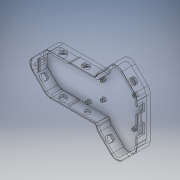
# Autodesk Inventor part: Arduino simple 4 channel ttl bottom Mega
Saved by Autodesk Inventor 2017 (Build 210142000, 142)
## iProperties
Created: 2016-10-03
Part Number: Arduino simple 4 channel ttl bottom Mega
Material: Generic
Document SubType Name: Modeling
Designer: andrew
Density: 1 g/cm^3
Appearance: Default
Author: andrew
Autodesk Inventor part; units mm, degrees
(part 1 of 2)
ref_plane "YZ Plane" through (0, 0, 0) normal (1, 0, 0) x (0, 1, 0)
ref_plane "XZ Plane" through (0, 0, 0) normal (0, 1, 0) x (-1, 0, 0)
ref_plane "XY Plane" through (0, 0, 0) normal (0, 0, 1) x (1, 0, 0)
sketch "Sketch1" plane through (0, 0, 0) normal (0, 1, 0) x (-1, 0, 0)
  circle A0 centre (66.1, -35.5) radius 2.345
  circle A1 centre (15.3, -50.7) radius 2.345
  circle A2 centre (14, -2.5) radius 2.345
  circle A3 centre (66.1, -7.6) radius 2.345
  line L0 (0, 0) -> (68.6, 0) construction
  line L1 (0, -53.3) -> (0, 0) construction
  line L2 (66.1, -53.3) -> (0, -53.3) construction
  line L3 (66.1, -40.6) -> (66.1, -53.3) construction
  line L4 (68.6, -40.6) -> (66.1, -40.6) construction
  line L5 (68.6, 0) -> (68.6, -40.6) construction
  line L6 (0, -12.2) -> (0, -3.3) construction
  line L7 (-1.8, -3.3) -> (0, -3.3) construction
  line L8 (-1.8, -12.2) -> (-1.8, -3.3) construction
  line L9 (0, -12.2) -> (-1.8, -12.2) construction
  line L10 (-6.2, -43.5895) -> (-6.2, -31.5895) construction
  line L11 (0, -43.5895) -> (0, -31.5895) construction
  line L12 (-6.2, -31.5895) -> (0, -31.5895) construction
  line L13 (-6.2, -43.5895) -> (-6.2, -31.5895) construction
  line L14 (0, -43.5895) -> (-6.2, -43.5895) construction
  circle A4 centre (14, -2.5) radius 1.6
  circle A5 centre (15.3, -50.7) radius 1.6
  circle A6 centre (66.1, -35.5) radius 1.6
  circle A7 centre (66.1, -7.6) radius 1.6
  line L15 (66.1, -35.5) -> (90.2, -35.5) construction
  line L16 (14, -2.5) -> (-6.2, -2.5) construction
  line L17 (0, -2.5) -> (96.52, -2.5) construction
  line L18 (0, -2.5) -> (96.52, -2.5) construction
  line L19 (90.2, -35.5) -> (90.2, -50.7) construction
  circle A8 centre (90.2, -50.7) radius 1.6
  circle A9 centre (90.2, -50.7) radius 2.345
  circle A10 centre (96.52, -2.5) radius 1.6
  circle A11 centre (96.52, -2.5) radius 2.345
  line L20 (68.6, -20.3) -> (101.6, -20.3) construction
  line L21 (101.6, -20.3) -> (101.6, 10.1637) construction
  dimension "d223" = 14
  dimension "d224" = 66.1
  dimension "d225" = 2.5
  dimension "d226" = 7.6
  dimension "d227" = 35.5
  dimension "d228" = 50.7
  dimension "d229" = 24.1
  dimension "d230" = 96.52
  dimension "d231" = 0
  dimension "d232" = 15.2
  dimension "d234" = 33
  constraints: 44 end point, 12 centre point, 4 horizontal, 2 collinear, 2 point on line, 2 vertical, 1 midpoint
  measures "d223" distance from line of L1 L16.start
  measures "d224" distance from line of A7.centre L1
  measures "d225" distance from line of L0 A2.centre
  measures "d226" distance from line of L0 A7.centre
  measures "d227" distance from line of L0 A0.centre
  measures "d228" distance from line of L0 A5.centre
  measures "d229" distance of L15.start L15.end
  measures "d230" distance of L17.start L17.end
  measures "d231" distance between parallel lines of L17 L18
  measures "d232" distance of L15.end L19.end
  measures "d234" distance of L20.start L20.end
extrude "Extrusion1" add sketch "Sketch1" along normal blind 4.69
draft "FaceDraft1" angle 10 pull direction (0, -1, 0) faces at (-68.4146, 3.1267, -7.9762) (-64.2253, 3.1267, -36.9087) (-16.3146, 3.1267, -2.8762) (-17.6146, 3.1267, -51.0762) (-98.8346, 3.1267, -2.8762) (-92.5146, 3.1267, -51.0762) fixed edges at (-63.755, 0, -7.6) (-63.755, 0, -35.5) (-11.655, 0, -2.5) (-12.955, 0, -50.7) (-94.175, 0, -2.5) (-87.855, 0, -50.7)
sketch "Sketch2" plane through (-66.1, 4.69, -7.6) normal (0, 1, 0) x (1, 0, 0)
  circle A0 centre (0.0002, 27.8999) radius 2.345 construction
  circle A1 centre (50.8002, 43.0999) radius 2.345 construction
  circle A2 centre (52.1002, -5.1001) radius 2.345 construction
  circle A3 centre (0.0002, -0.0001) radius 2.345 construction
  line L0 (66.1002, -7.6001) -> (-2.4998, -7.6001) construction
  line L1 (66.1002, 45.6999) -> (66.1002, -7.6001) construction
  line L2 (0.0002, 45.6999) -> (66.1002, 45.6999) construction
  line L3 (0.0002, 32.9999) -> (0.0002, 45.6999) construction
  line L4 (-2.4998, 32.9999) -> (0.0002, 32.9999) construction
  line L5 (-2.4998, -7.6001) -> (-2.4998, 32.9999) construction
  line L6 (66.1002, 4.5999) -> (66.1002, -4.3001) construction
  line L7 (67.9002, -4.3001) -> (66.1002, -4.3001) construction
  line L8 (66.1002, 4.5999) -> (67.9002, 4.5999) construction
  line L9 (72.3002, 35.9894) -> (72.3002, 23.9894) construction
  line L10 (66.1002, 35.9894) -> (66.1002, 23.9894) construction
  line L11 (72.3002, 23.9894) -> (66.1002, 23.9894) construction
  line L12 (72.3002, 35.9894) -> (72.3002, 23.9894) construction
  line L13 (66.1002, 35.9894) -> (72.3002, 35.9894) construction
  circle A4 centre (52.1002, -5.1001) radius 1.6 construction
  circle A5 centre (50.8002, 43.0999) radius 1.6 construction
  circle A6 centre (0.0002, 27.8999) radius 1.6 construction
  circle A7 centre (0.0002, -0.0001) radius 1.6 construction
  line L14 (-4.4998, -9.6001) -> (68.1002, -9.6001) construction
  line L15 (-1.9998, 47.6999) -> (-1.9998, 34.9999) construction
  line L16 (-1.9998, 34.9999) -> (-4.4998, 34.9999) construction
  line L17 (66.1002, 4.5999) -> (74.6809, 4.5999) construction
  line L18 (74.6809, 4.5999) -> (74.6809, -4.3001) construction
  line L19 (74.6809, -4.3001) -> (66.1002, -4.3001) construction
  line L20 (66.1002, -4.3001) -> (66.1002, 4.5999) construction
  line L21 (66.1002, 23.9894) -> (80.0982, 23.9894) construction
  line L22 (80.0982, 23.9894) -> (80.0982, 35.9894) construction
  line L23 (80.0982, 35.9894) -> (66.1002, 35.9894) construction
  line L24 (66.1002, 35.9894) -> (66.1002, 23.9894) construction
  line L25 (76.0853, 6.0043) -> (64.6958, 6.0043) construction
  line L26 (64.6958, 6.0043) -> (64.6958, -5.7045) construction
  line L27 (64.6958, -5.7045) -> (76.0853, -5.7045) construction
  line L28 (76.0853, -5.7045) -> (76.0853, 6.0043) construction
  line L29 (82.0982, 21.9894) -> (64.1002, 21.9894) construction
  line L30 (64.1002, 21.9894) -> (64.1002, 37.9894) construction
  line L31 (64.1002, 37.9894) -> (82.0982, 37.9894) construction
  line L32 (82.0982, 37.9894) -> (82.0982, 21.9894) construction
  line L33 (68.1002, 6.0043) -> (71.1002, 6.0043)
  line L34 (71.1002, 21.9894) -> (68.1002, 21.9894)
  line L35 (71.1002, 37.9894) -> (68.1002, 37.9894) construction
  line L36 (68.1002, 6.0043) -> (68.1002, 47.6999) construction
  line L37 (68.1002, 47.6999) -> (68.1002, 37.9894) construction
  line L38 (68.1002, 21.9894) -> (68.1002, 6.0043)
  line L39 (71.1002, 37.9894) -> (71.1002, 50.6999) construction
  line L40 (68.1002, -9.6001) -> (68.1002, -10.3919) construction
  line L41 (68.1002, 47.6999) -> (68.1002, 49.1999) construction
  line L42 (68.1002, 47.6999) -> (69.6002, 47.6999) construction
  line L43 (71.1002, 50.6999) -> (71.1002, 52.1999) construction
  line L44 (71.1002, 50.6999) -> (72.6002, 50.6999) construction
  line L45 (6.3002, -11.1001) -> (-38.5071, -11.1001)
  line L46 (71.1002, -14.1001) -> (71.1002, -5.7045) construction
  line L47 (71.1002, 6.0043) -> (71.1002, 21.9894)
  line L48 (71.1002, -5.7045) -> (68.1002, -5.7045) construction
  line L49 (-74.3828, 65.0749) -> (-74.3828, 33.3249) construction
  line L50 (-62.8828, 49.1999) -> (-62.8828, 33.3249) construction
  line L51 (-67.8378, 49.1999) -> (-62.8828, 49.1999) construction
  line L52 (-67.8378, 33.3249) -> (-67.8378, 65.0749) construction
  line L53 (-74.3828, 33.3249) -> (-61.2928, 33.3249) construction
  line L54 (-74.3828, 49.1999) -> (-61.2928, 49.1999) construction
  line L55 (-68.9958, 47.6999) -> (-42.4924, 47.6999)
  line L56 (-62.8828, 33.3249) -> (-72.7928, 33.3249) construction
  line L57 (-86.1418, 1.9038) -> (-89.6456, 5.4076) construction
  line L58 (-89.6456, 5.4076) -> (-78.4202, 16.6329) construction
  line L59 (-78.4202, 16.6329) -> (-71.4128, 9.6254) construction
  line L60 (-79.5445, 17.7572) -> (-70.2885, 8.5011) construction
  line L61 (-101.9952, -4.6935) -> (-79.5445, 17.7572) construction
  line L62 (-90.7699, 6.5319) -> (-81.5138, -2.7242) construction
  line L63 (-71.4128, 9.6254) -> (-82.6381, -1.5999) construction
  line L64 (-75.0062, -7.1105) -> (-95.1562, 13.0395)
  line L65 (-74.9165, 13.1292) -> (-97.3672, -9.3215) construction
  line L66 (-78.1882, -10.2925) -> (-98.3382, 9.8575)
  line L67 (-70.2885, 8.5011) -> (-92.7391, -13.9495) construction
  line L68 (-92.7391, -13.9495) -> (-101.9952, -4.6935) construction
  arc A8 (-98.3382, 28.2423) -> (-98.3382, 9.8575) centre (-89.1458, 19.0499) ccw
  arc A9 (-95.1562, 25.0603) -> (-95.1562, 13.0395) centre (-89.1458, 19.0499) ccw
  line L69 (-42.4924, -9.6001) -> (-68.9958, -9.6001)
  arc A10 (-75.0062, -7.1105) -> (-68.9958, -9.6001) centre (-68.9958, -1.1001) ccw
  arc A11 (-78.1882, -10.2925) -> (-68.9958, -14.1001) centre (-68.9958, -1.1001) ccw
  line L70 (-61.2928, 33.3249) -> (-61.2928, 65.0749) construction
  line L71 (-72.7928, 33.3249) -> (-72.7928, 49.1999) construction
  arc A12 (-68.9958, 47.6999) -> (-75.0062, 45.2103) centre (-68.9958, 39.1999) ccw
  arc A13 (-68.9958, 52.1999) -> (-78.1882, 48.3923) centre (-68.9958, 39.1999) ccw
  line L72 (-98.3382, 28.2423) -> (-78.1882, 48.3923)
  line L73 (-95.1562, 25.0603) -> (-75.0062, 45.2103)
  line L74 (-40.4998, -10.3501) -> (-40.4998, -10.3501)
  line L75 (-40.4998, 48.4499) -> (-40.4998, 48.4499)
  line L76 (-40.3711, -10.4788) -> (-40.6284, -10.2214)
  line L77 (-40.3711, 48.5786) -> (-39.7498, 49.1999)
  line L78 (-85.0812, 2.9645) -> (-92.329, 10.2123) construction
  line L79 (-92.329, 10.2123) -> (-92.329, 27.8875) construction
  line L80 (-35.4998, 19.0499) -> (-68.4998, 19.0499) construction
  line L81 (8.5832, -108.4404) -> (8.5832, -95.3504) construction
  line L82 (8.5832, -106.8504) -> (-7.2918, -106.8504) construction
  line L83 (8.5832, -96.9404) -> (8.5832, -106.8504) construction
  arc A14 (49.0186, -109.0638) -> (51.5082, -103.0534) centre (43.0082, -103.0534) ccw
  arc A15 (52.2006, -112.2458) -> (56.0082, -103.0534) centre (43.0082, -103.0534) ccw
  line L84 (31.1405, -104.3283) -> (42.3658, -115.5537) construction
  line L85 (24.1331, -111.3358) -> (31.1405, -104.3283) construction
  line L86 (23.0088, -112.4601) -> (32.2648, -103.204) construction
  line L87 (32.2648, -103.204) -> (54.7155, -125.6547) construction
  line L88 (38.8621, -119.0574) -> (35.3584, -122.5611) construction
  line L89 (34.2341, -123.6854) -> (43.4901, -114.4294) construction
  line L90 (35.3584, -122.5611) -> (24.1331, -111.3358) construction
  line L91 (49.0186, -109.0638) -> (28.8686, -129.2138)
  line L92 (27.6368, -107.832) -> (50.0874, -130.2827) construction
  line L93 (52.2006, -112.2458) -> (32.0506, -132.3958)
  line L94 (45.4594, -134.9107) -> (23.0088, -112.4601) construction
  arc A16 (16.8478, -129.2138) -> (28.8686, -129.2138) centre (22.8582, -123.2034) ccw
  arc A17 (13.6658, -132.3958) -> (32.0506, -132.3958) centre (22.8582, -123.2034) ccw
  line L95 (16.8478, -129.2138) -> (-3.3022, -109.0638)
  line L96 (13.6658, -132.3958) -> (-6.4842, -112.2458)
  line L97 (54.7155, -125.6547) -> (45.4594, -134.9107) construction
  line L98 (-7.2918, -108.4404) -> (-7.2918, -95.3504) construction
  line L99 (-23.1668, -108.4404) -> (8.5832, -108.4404) construction
  arc A18 (-5.7918, -103.0534) -> (-3.3022, -109.0638) centre (2.7082, -103.0534) ccw
  arc A19 (-10.2918, -103.0534) -> (-6.4842, -112.2458) centre (2.7082, -103.0534) ccw
  line L100 (38.9436, -119.1388) -> (31.6958, -126.3867) construction
  line L101 (31.6958, -126.3867) -> (14.0206, -126.3867) construction
  line L102 (53.9542, -30.104) -> (50.4504, -33.6077) construction
  line L103 (49.3261, -34.732) -> (58.5822, -25.476) construction
  line L104 (50.4504, -33.6077) -> (39.2251, -22.3824) construction
  line L105 (39.2251, -22.3824) -> (46.2326, -15.375) construction
  line L106 (38.1008, -23.5067) -> (47.3569, -14.2507) construction
  line L107 (60.5515, -45.9574) -> (38.1008, -23.5067) construction
  line L108 (69.8075, -36.7013) -> (60.5515, -45.9574) construction
  line L109 (67.2926, -23.2925) -> (47.1426, -43.4425)
  line L110 (64.1106, -20.1105) -> (43.9606, -40.2605)
  line L111 (42.7288, -18.8787) -> (65.1795, -41.3293) construction
  line L112 (47.3569, -14.2507) -> (69.8075, -36.7013) construction
  arc A20 (64.1106, -20.1105) -> (66.5817, -14.6605) centre (58.1002, -14.1001) ccw construction
  arc A21 (67.2926, -23.2925) -> (71.1002, -14.1001) centre (58.1002, -14.1001) ccw construction
  line L113 (46.2326, -15.375) -> (57.4579, -26.6003) construction
  arc A22 (31.9398, -40.2605) -> (43.9606, -40.2605) centre (37.9502, -34.2501) ccw
  arc A23 (28.7578, -43.4425) -> (47.1426, -43.4425) centre (37.9502, -34.2501) ccw
  line L114 (46.7878, -37.4333) -> (29.1127, -37.4333) construction
  line L115 (23.6752, -19.4871) -> (23.6752, -6.3971) construction
  line L116 (23.6752, -17.8971) -> (7.8002, -17.8971) construction
  line L117 (23.6752, -7.9871) -> (23.6752, -17.8971) construction
  line L118 (31.9398, -40.2605) -> (11.7898, -20.1105)
  line L119 (28.7578, -43.4425) -> (8.6078, -23.2925)
  arc A24 (9.3002, -14.1001) -> (11.7898, -20.1105) centre (17.8002, -14.1001) ccw
  arc A25 (5.0308, -16.5376) -> (8.6078, -23.2925) centre (17.8002, -14.1001) ccw
  line L120 (7.8002, -19.4871) -> (7.8002, -6.3971) construction
  line L121 (-8.0748, -19.4871) -> (23.6752, -19.4871) construction
  line L122 (54.0356, -30.1855) -> (46.7878, -37.4333) construction
  line L123 (-68.9958, -14.1001) -> (2.084, -14.1001)
  line L124 (9.3002, -14.1001) -> (9.3002, -14.1001)
  arc A26 (5.0308, -16.5376) -> (2.084, -14.1001) centre (2.084, -17.1001) ccw
  arc A27 (9.3002, -14.1001) -> (6.3002, -11.1001) centre (6.3002, -14.1001) ccw
  arc A28 (-40.6284, -10.2214) -> (-38.5071, -11.1001) centre (-38.5071, -8.1001) ccw
  arc A29 (-40.3711, -10.4788) -> (-42.4924, -9.6001) centre (-42.4924, -12.6001) ccw
  arc A30 (-42.4924, 47.6999) -> (-40.3711, 48.5786) centre (-42.4924, 50.6999) ccw
  line L125 (-16.5053, 19.0499) -> (-10.8424, 19.0499) construction
  line L126 (71.1002, 52.1999) -> (71.1002, 43.8043) construction
  line L127 (53.9542, 68.2038) -> (50.4504, 71.7076) construction
  line L128 (50.4504, 71.7076) -> (39.2251, 60.4822) construction
  line L129 (39.2251, 60.4822) -> (46.2326, 53.4748) construction
  line L130 (38.1008, 61.6065) -> (47.3569, 52.3505) construction
  line L131 (54.0356, 68.2853) -> (46.7878, 75.5332) construction
  line L132 (46.2326, 53.4748) -> (57.4579, 64.7001) construction
  line L133 (49.3261, 72.8319) -> (58.5822, 63.5758) construction
  line L134 (60.5515, 84.0572) -> (38.1008, 61.6065) construction
  line L135 (47.3569, 52.3505) -> (69.8075, 74.8011) construction
  line L136 (69.8075, 74.8011) -> (60.5515, 84.0572) construction
  line L137 (67.2926, 61.3923) -> (47.1426, 81.5423)
  line L138 (42.7288, 56.9785) -> (65.1795, 79.4292) construction
  line L139 (64.1106, 58.2103) -> (43.9606, 78.3603)
  arc A31 (66.5817, 52.7604) -> (64.1106, 58.2103) centre (58.1002, 52.1999) ccw construction
  arc A32 (71.1002, 52.1999) -> (67.2926, 61.3923) centre (58.1002, 52.1999) ccw construction
  line L140 (31.9398, 78.3603) -> (11.7898, 58.2103)
  line L141 (28.7578, 81.5423) -> (8.6078, 61.3923)
  line L142 (23.6752, 46.0869) -> (23.6752, 55.9969) construction
  line L143 (23.6752, 57.5869) -> (23.6752, 44.4969) construction
  line L144 (23.6752, 55.9969) -> (7.8002, 55.9969) construction
  arc A33 (11.7898, 58.2103) -> (9.3002, 52.1999) centre (17.8002, 52.1999) ccw
  arc A34 (8.6078, 61.3923) -> (5.0308, 54.6374) centre (17.8002, 52.1999) ccw
  line L145 (7.8002, 57.5869) -> (7.8002, 44.4969) construction
  line L146 (-8.0748, 57.5869) -> (23.6752, 57.5869) construction
  arc A35 (43.9606, 78.3603) -> (31.9398, 78.3603) centre (37.9502, 72.3499) ccw
  arc A36 (47.1426, 81.5423) -> (28.7578, 81.5423) centre (37.9502, 72.3499) ccw
  line L147 (46.7878, 75.5332) -> (29.1127, 75.5332) construction
  line L148 (9.3002, 52.1999) -> (9.3002, 52.1999)
  arc A37 (2.084, 52.1999) -> (5.0308, 54.6374) centre (2.084, 55.1999) ccw
  arc A38 (6.3002, 49.1999) -> (9.3002, 52.1999) centre (6.3002, 52.1999) ccw
  arc A39 (66.5817, 52.7604) -> (66.8919, 51.6165) centre (69.5752, 52.9582) ccw construction
  line L149 (6.3002, 49.1999) -> (-39.7498, 49.1999)
  line L150 (-68.9958, 52.1999) -> (2.084, 52.1999)
  line L151 (66.8919, 51.6165) -> (68.1002, 49.1999) construction
  line L152 (66.5817, -14.6605) -> (68.1002, -10.3919) construction
  line L153 (66.5817, -14.6605) -> (68.1002, -10.3919)
  line L154 (68.1002, -10.3919) -> (68.1002, -5.7045)
  line L155 (68.1002, -5.7045) -> (71.1002, -5.7045)
  line L156 (71.1002, -5.7045) -> (71.1002, -14.1001)
  arc A40 (67.2926, -23.2925) -> (71.1002, -14.1001) centre (58.1002, -14.1001) ccw
  arc A41 (64.1106, -20.1105) -> (66.5817, -14.6605) centre (58.1002, -14.1001) ccw
  line L157 (71.1002, 52.1999) -> (71.1002, 37.9894)
  line L158 (71.1002, 37.9894) -> (68.1002, 37.9894)
  line L159 (68.1002, 37.9894) -> (68.1002, 49.1999)
  line L160 (68.1002, 49.1999) -> (66.8919, 51.6165)
  arc A42 (66.8919, 51.6165) -> (64.1106, 58.2103) centre (57.0713, 51.3576) ccw
  arc A43 (71.1002, 52.1999) -> (67.2926, 61.3923) centre (58.1002, 52.1999) ccw
  point P0 (66.1, -7.6)
  point P1 (66.1002, -7.6001)
  point P2 (-73.1379, -11.1001)
  point P3 (-103.2879, 19.0499)
  point P4 (53.0082, -107.1956)
  point P5 (22.8582, -137.3456)
  point P6 (68.1002, -18.2422)
  point P7 (66.6002, -14.1001)
  point P8 (37.9502, -48.3922)
  point P9 (4.8002, -14.1001)
  point P10 (37.9502, 86.492)
  point P11 (66.6002, 52.1999)
  point P12 (68.1002, 56.342)
  point P13 (4.8002, 52.1999)
  point P14 (-12.4473, 49.1999)
  point P15 (-12.4473, 52.1999)
  point P16 (-8.5418, -11.1001)
  point P17 (-8.5418, -14.1001)
  dimension "d7" = 2
  dimension "d9" = 2
  dimension "d53" = 1.5
  dimension "d54" = 90
  dimension "d55" = 1.5
  dimension "d56" = 90
  dimension "d146" = 4.955
  dimension "d147" = 9.91
  dimension "d152" = 31.75
  dimension "d153" = 13.09
  dimension "d154" = 4.955
  dimension "d155" = 9.91
  dimension "d204" = 10.25
  dimension "d205" = 17.6751
  dimension "d237" = 33
  dimension "d238" = 4.955
  dimension "d239" = 9.91
  dimension "d240" = 13.09
  dimension "d241" = 9.91
  dimension "d242" = 10.25
  dimension "d243" = 17.6751
  dimension "d244" = 4.955
  dimension "d245" = 9.91
  dimension "d246" = 13.09
  dimension "d247" = 9.91
  dimension "d248" = 10.25
  dimension "d249" = 17.6751
  dimension "d250" = 3
  constraints: 322 end point, 76 point on circle, 54 point on line, 50 symmetric about line, 44 centre point, 25 midpoint, 25 perpendicular, 15 parallel, 12 tangent, 10 horizontal, 7 vertical, 5 equal radius, 4 collinear, 1 coincident, 27 other
  measures "d7" distance between parallel lines of L0 L14
  measures "d9" distance between parallel lines of L21 L29
  measures "d53" distance of L36.end L41.end
  measures "d54" angle of L42 L41
  measures "d55" distance of L43.end L39.end
  measures "d56" angle of L44 L43
  measures "d146" distance of L57.start L57.end
  measures "d147" distance of L59.start L63.start
  measures "d152" distance of L53.end L70.end
  measures "d153" distance of L53.start L53.end
  measures "d154" distance of L51.start L50.start
  measures "d155" distance of L56.start L71.start
  measures "d204" distance of L78.start L78.end
  measures "d205" distance of L78.end L79.end
  measures "d237" distance of L80.start L80.end
  measures "d238" distance of L88.start L88.end
  measures "d239" distance of L90.end L85.end
  measures "d240" distance of L81.start L81.end
  measures "d241" distance of L83.start L82.start
  measures "d242" distance of L100.start L101.start
  measures "d243" distance of L101.start L101.end
  measures "d244" distance of L102.start L102.end
  measures "d245" distance of L104.end L105.end
  measures "d246" distance of L115.start L115.end
  measures "d247" distance of L117.start L117.end
  measures "d248" distance of L122.start L122.end
  measures "d249" distance of L122.end L114.end
  measures "d250" radius of A26
extrude "Extrusion2" add sketch "Sketch2" against normal blind 17.29
sketch "Sketch4" plane through (-66.1, -12.6, -7.6) normal (0, -1, 0) x (1, 0, 0)
  line L0 (-118.6267, 83.4161) -> (-86.8767, 83.4161)
  line L1 (-86.8767, 83.4161) -> (-86.8767, 70.3261)
  line L2 (-86.8767, 70.3261) -> (-118.6267, 70.3261)
  line L3 (-118.6267, 70.3261) -> (-118.6267, 83.4161)
  line L4 (-86.8767, 76.8711) -> (-118.6267, 76.8711)
  line L5 (-102.7517, 83.4161) -> (-102.7517, 70.3261)
  line L6 (-102.7517, 76.8711) -> (-102.7517, 81.8261)
  line L7 (-102.7517, 81.8261) -> (-86.8767, 81.8261)
  line L8 (-86.8767, 81.8261) -> (-86.8767, 71.9161)
  line L9 (-86.8767, 71.9161) -> (-102.7517, 71.9161)
  line L10 (-118.7515, 30.5625) -> (-96.3008, 53.0132)
  line L11 (-96.3008, 53.0132) -> (-87.0448, 43.7571)
  line L12 (-87.0448, 43.7571) -> (-109.4954, 21.3065)
  line L13 (-109.4954, 21.3065) -> (-118.7515, 30.5625)
  line L14 (-91.6728, 48.3851) -> (-114.1234, 25.9345)
  line L15 (-107.5261, 41.7878) -> (-98.2701, 32.5318)
  line L16 (-102.8981, 37.1598) -> (-106.4018, 40.6635)
  line L17 (-106.4018, 40.6635) -> (-95.1765, 51.8889)
  line L18 (-95.1765, 51.8889) -> (-88.1691, 44.8814)
  line L19 (-88.1691, 44.8814) -> (-99.3944, 33.6561)
  line L20 (-89.2658, 116.7338) -> (-66.8151, 94.2832)
  line L21 (-66.8151, 94.2832) -> (-76.0711, 85.0271)
  line L22 (-76.0711, 85.0271) -> (-98.5218, 107.4778)
  line L23 (-98.5218, 107.4778) -> (-89.2658, 116.7338)
  line L24 (-71.4431, 89.6551) -> (-93.8938, 112.1058)
  line L25 (-78.0404, 105.5085) -> (-87.2965, 96.2524)
  line L26 (-82.6685, 100.8805) -> (-79.1647, 104.3842)
  line L27 (-79.1647, 104.3842) -> (-67.9394, 93.1589)
  line L28 (-67.9394, 93.1589) -> (-74.9468, 86.1514)
  line L29 (-74.9468, 86.1514) -> (-86.1722, 97.3767)
  line L30 (71.1002, -52.1999) -> (-7.4998, -52.1999)
  line L31 (-7.4998, -52.1999) -> (-7.4998, 14.1001)
  line L32 (-7.4998, 14.1001) -> (71.1002, 14.1001)
  line L33 (71.1002, 14.1001) -> (71.1002, -52.1999)
  line L34 (68.1002, 11.1001) -> (68.1002, 5.7045) projected
  line L35 (68.1002, -49.1999) -> (-39.7498, -49.1999) projected
  line L36 (68.1002, 11.1001) -> (-4.4998, 11.1001)
  line L37 (-4.4998, 11.1001) -> (-4.4998, -49.1999)
  line L38 (-4.4998, -49.1999) -> (68.1002, -49.1999)
  line L39 (68.1002, -49.1999) -> (68.1002, 11.1001)
  line L40 (-4.4998, -49.1999) -> (34.0716, -49.1999) construction
  line L41 (-7.4998, 14.1001) -> (-7.4998, -52.1999) projected
  line L42 (-7.4998, -19.0499) -> (35.1392, -19.0499) construction
  line L43 (-7.4998, 14.1001) -> (-7.4998, -52.1999)
  line L44 (-101.9952, -42.7933) -> (-79.5445, -20.3426) construction
  line L45 (-79.5445, -20.3426) -> (-70.2885, -29.5987) construction
  line L46 (-70.2885, -29.5987) -> (-92.7391, -52.0493) construction
  line L47 (-71.4128, -28.4744) -> (-82.6381, -39.6997) construction
  line L48 (-74.9165, -24.9707) -> (-97.3672, -47.4213) construction
  line L49 (-92.7391, -52.0493) -> (-101.9952, -42.7933)
  line L50 (-86.1418, -36.196) -> (-89.6456, -32.6923) construction
  line L51 (-90.7699, -31.568) -> (-81.5138, -40.824) construction
  line L52 (-78.4202, -21.4669) -> (-71.4128, -28.4744) construction
  line L53 (-89.6456, -32.6923) -> (-78.4202, -21.4669) construction
  line L54 (-91.8047, 14.9002) -> (-69.3541, -7.5505) construction
  line L55 (-69.3541, -7.5505) -> (-78.6101, -16.8065) construction
  line L56 (-78.6101, -16.8065) -> (-101.0607, 5.6441) construction
  line L57 (-101.0607, 5.6441) -> (-91.8047, 14.9002)
  line L58 (-73.9821, -12.1785) -> (-96.4327, 10.2722) construction
  line L59 (-77.4858, -15.6822) -> (-88.7111, -4.4569) construction
  line L60 (-85.2074, -0.9532) -> (-81.7037, 2.5506)
  line L61 (-81.7037, 2.5506) -> (-70.4784, -8.6748) construction
  line L62 (-70.4784, -8.6748) -> (-77.4858, -15.6822) construction
  line L63 (-80.5794, 3.6749) -> (-89.8354, -5.5812) construction
  line L64 (-15.2028, 26.9751) -> (-15.2028, -4.7749) construction
  line L65 (-48.2028, -4.7749) -> (-61.2928, -4.7749) construction
  line L66 (-61.2928, -4.7749) -> (-61.2928, 26.9751) construction
  line L67 (-61.2928, 26.9751) -> (-48.2028, 26.9751) construction
  line L68 (-21.7478, -4.7749) -> (-21.7478, 26.9751) construction
  line L69 (-16.7928, 11.1001) -> (-16.7928, -4.7749) construction
  line L70 (-21.7478, 11.1001) -> (-16.7928, 11.1001) construction
  line L71 (-49.7928, -4.7749) -> (-59.7028, -4.7749) construction
  line L72 (-59.7028, -4.7749) -> (-59.7028, 11.1001) construction
  line L73 (-48.2028, 11.1001) -> (-61.2928, 11.1001) construction
  line L74 (-4.4998, 11.1001) -> (-7.4998, 11.1001)
  line L75 (-40.4998, -52.1999) -> (-68.9958, -52.1999)
  arc A0 (-78.1882, -48.3923) -> (-68.9958, -52.1999) centre (-68.9958, -39.1999) ccw
  line L76 (-78.1882, -48.3923) -> (-98.3382, -28.2423)
  arc A1 (-98.3382, -9.8575) -> (-98.3382, -28.2423) centre (-89.1458, -19.0499) ccw
  line L77 (-98.3382, -9.8575) -> (-78.1882, 10.2924)
  arc A2 (-68.9958, 14.1001) -> (-78.1882, 10.2924) centre (-68.9957, 1.1) ccw
  line L78 (-68.9958, 14.1001) -> (-40.4998, 14.1004)
  line L79 (-40.4998, -47.6999) -> (-68.9958, -47.6999)
  arc A3 (-75.0062, -45.2103) -> (-68.9958, -47.6999) centre (-68.9958, -39.1999) ccw
  line L80 (-75.0062, -45.2103) -> (-95.1562, -25.0603)
  arc A4 (-95.1562, -13.0395) -> (-95.1562, -25.0603) centre (-89.1458, -19.0499) ccw
  line L81 (-95.1562, -13.0395) -> (-75.0062, 7.1105)
  arc A5 (-68.9957, 9.6001) -> (-75.0062, 7.1105) centre (-68.9957, 1.1) ccw
  line L82 (-68.9957, 9.6001) -> (-40.4997, 9.6004)
  line L83 (57.13, 22.4364) -> (24.13, 22.4364) construction
  point P0 (-103.2879, -19.0499)
  point P1 (-73.1379, -49.1999)
  dimension "d12" = 31.75
  dimension "d13" = 13.09
  dimension "d14" = 4.955
  dimension "d15" = 9.91
  dimension "d34" = 13.09
  dimension "d35" = 4.955
  dimension "d36" = 9.91
  dimension "d42" = 31.75
  dimension "d43" = 13.09
  dimension "d44" = 4.955
  dimension "d45" = 9.91
  dimension "d92" = 42.6385
  dimension "d102" = 13.09
  dimension "d103" = 4.955
  dimension "d104" = 9.91
  dimension "d105" = 31.75
  dimension "d106" = 13.09
  dimension "d107" = 4.955
  dimension "d108" = 9.91
  dimension "d111" = 31.75
  dimension "d112" = 13.09
  dimension "d113" = 4.955
  dimension "d114" = 9.91
  dimension "d117" = 4.5
  dimension "d235" = 33
  constraints: 162 end point, 27 midpoint, 24 point on line, 21 perpendicular, 17 equal length, 12 point on circle, 6 centre point, 6 horizontal, 6 other
  measures "d12" distance of L1.end L2.end
  measures "d13" distance of L0.end L1.end
  measures "d14" distance of L6.start L6.end
  measures "d15" distance of L7.end L8.end
  measures "d34" distance of L10.end L11.end
  measures "d35" distance of L16.start L16.end
  measures "d36" distance of L18.start L19.start
  measures "d42" distance of L21.end L22.end
  measures "d43" distance of L20.end L21.end
  measures "d44" distance of L26.start L26.end
  measures "d45" distance of L27.end L29.start
  measures "d92" distance of point (-73.138, -49.2) point (-103.288, -19.05)
  measures "d102" distance of L45.start L45.end
  measures "d103" distance of L50.start L53.start
  measures "d104" distance of L52.start L52.end
  measures "d105" distance of L55.end L57.start
  measures "d106" distance of L55.start L55.end
  measures "d107" distance of L60.start L60.end
  measures "d108" distance of L62.start L59.start
  measures "d111" distance of L65.end L66.end
  measures "d112" distance of L65.start L65.end
  measures "d113" distance of L70.start L69.start
  measures "d114" distance of L71.start L71.end
  measures "d117" radial gap between concentric circles of A2 A5
  measures "d235" distance of L83.start L83.end
fillet "Fillet1" radius 2 1 edges at (-105.8498, -3.955, -56.7999)
sketch "Sketch6" plane through (-144.2882, -12.6, -55.9923) normal (-0.7071068, 0, -0.7071068) x (-0.7071068, 0, 0.7071068)
  arc A0 (12.3053, 11.18) -> (18.6412, 11.18) centre (15.4732, 7.37) ccw
  line L0 (12.3053, 11.18) -> (18.6412, 11.18)
  line L1 (15.4732, 8.37) -> (15.4732, 7.37)
  line L2 (15.4732, 8.37) -> (16.4732, 8.37) construction
  line L3 (0, 17.29) -> (28.4964, 17.29) projected
  line L4 (15.4732, 17.29) -> (15.4732, 11.18)
  line L5 (15.4732, 11.18) -> (15.4732, 10.2293)
  point P0 (-62.4346, 12.6)
  point P1 (28.4964, 16)
  dimension "d164" = 9.91
  dimension "d188" = 1
  dimension "d189" = 90
  dimension "d337" = 6.11
  dimension "d338" = 6.11
  constraints: 10 end point, 2 horizontal, 2 point on circle, 1 centre point, 1 midpoint, 1 perpendicular, 1 vertical
  measures "d164" diameter of A0
  measures "d188" distance of L1.start L1.end
  measures "d189" angle of L1 L2
  measures "d337" distance between parallel lines of L3 L0
  measures "d338" distance of L4.start L4.end
extrude "Extrusion4" cut sketch "Sketch6" against normal blind 10
sketch "Sketch7" plane through (-164.4382, -12.6, -17.4575) normal (-0.7071068, 0, 0.7071068) x (0.7071068, 0, 0.7071068)
  line L0 (28.4964, 8) -> (0, 8) construction
  line L1 (14.1948, 7) -> (14.1948, 0) construction
  arc A0 (11.1256, 10.89) -> (17.264, 10.89) centre (14.1948, 7) ccw
  line L2 (14.1948, 0) -> (14.1948, 17.29) projected
  line L3 (14.1948, 8) -> (18.0848, 8) construction
  line L4 (11.1256, 10.89) -> (17.264, 10.89)
  line L5 (14.1948, 14.245) -> (14.1948, 17.29)
  line L6 (21.1672, 8) -> (21.1672, 7)
  line L7 (21.1672, 8) -> (22.1672, 8) construction
  point P0 (128.6197, 12.6)
  dimension "d171" = 9.91
  dimension "d179" = 3.045
  dimension "d190" = 1
  dimension "d191" = 90
  constraints: 14 end point, 2 horizontal, 2 point on circle, 2 point on line, 1 centre point, 1 coincident, 1 collinear, 1 perpendicular, 1 vertical
  measures "d171" diameter of A0
  measures "d179" distance of L2.end L5.start
  measures "d190" distance of L6.start L6.end
  measures "d191" angle of L6 L7
extrude "Extrusion5" cut sketch "Sketch7" against normal blind 10
sketch "Sketch8" plane through (-66.1, 4.69, -7.6) normal (0, 1, 0) x (1, 0, 0)
  line L0 (6.3002, -11.1001) -> (-38.5071, -11.1001) projected
  line L1 (-40.6284, -10.2214) -> (-40.3711, -10.4788) projected
  line L2 (-42.4924, -9.6001) -> (-68.9958, -9.6001) projected
  arc A0 (-75.0062, -7.1105) -> (-68.9958, -9.6001) centre (-68.9958, -1.1001) ccw projected
  line L3 (-75.0062, -7.1105) -> (-95.1562, 13.0395) projected
  arc A1 (-95.1562, 25.0603) -> (-95.1562, 13.0395) centre (-89.1458, 19.0499) ccw projected
  line L4 (-95.1562, 25.0603) -> (-75.0062, 45.2103) projected
  arc A2 (-68.9958, 47.6999) -> (-75.0062, 45.2103) centre (-68.9958, 39.1999) ccw projected
  line L5 (-68.9958, 47.6999) -> (-42.4924, 47.6999) projected
  line L6 (-40.3711, 48.5786) -> (-40.3356, 48.6141) projected
  arc A3 (-38.9213, 49.1999) -> (-40.3356, 48.6141) centre (-38.9213, 47.1999) ccw projected
  arc A4 (-68.9958, 52.1999) -> (-78.1882, 48.3923) centre (-68.9958, 39.1999) ccw projected
  line L7 (-78.1882, 48.3923) -> (-98.3382, 28.2423) projected
  arc A5 (-98.3382, 28.2423) -> (-98.3382, 9.8575) centre (-89.1458, 19.0499) ccw projected
  line L8 (-98.3382, 9.8575) -> (-78.1882, -10.2925) projected
  arc A6 (-78.1882, -10.2925) -> (-68.9958, -14.1001) centre (-68.9958, -1.1001) ccw projected
  line L9 (71.1002, 37.9894) -> (71.1002, -5.7045)
  arc A7 (-42.4924, 47.6999) -> (-40.3711, 48.5786) centre (-42.4924, 50.6999) ccw projected
  line L10 (-38.9213, 49.1999) -> (6.3002, 49.1999) projected
  line L11 (2.084, 52.1999) -> (-68.9958, 52.1999) projected
  line L12 (-68.9958, -14.1001) -> (2.084, -14.1001) projected
  arc A8 (-40.6284, -10.2214) -> (-38.5071, -11.1001) centre (-38.5071, -8.1001) ccw projected
  arc A9 (-40.3711, -10.4788) -> (-42.4924, -9.6001) centre (-42.4924, -12.6001) ccw projected
  arc A10 (5.0308, -16.5376) -> (2.084, -14.1001) centre (2.084, -17.1001) ccw projected
  arc A11 (5.0308, -16.5376) -> (8.6078, -23.2925) centre (17.8002, -14.1001) ccw projected
  line L13 (8.6078, -23.2925) -> (28.7578, -43.4425) projected
  arc A12 (28.7578, -43.4425) -> (47.1426, -43.4425) centre (37.9502, -34.2501) ccw projected
  line L14 (47.1426, -43.4425) -> (67.2926, -23.2925) projected
  line L15 (64.1106, -20.1105) -> (43.9606, -40.2605) projected
  arc A13 (31.9398, -40.2605) -> (43.9606, -40.2605) centre (37.9502, -34.2501) ccw projected
  line L16 (31.9398, -40.2605) -> (11.7898, -20.1105) projected
  arc A14 (9.3002, -14.1001) -> (11.7898, -20.1105) centre (17.8002, -14.1001) ccw projected
  arc A15 (9.3002, -14.1001) -> (6.3002, -11.1001) centre (6.3002, -14.1001) ccw projected
  line L17 (68.1002, -5.7045) -> (68.1002, -10.3919) projected
  line L18 (68.1002, -10.3919) -> (66.5817, -14.6605) projected
  arc A16 (64.1106, -20.1105) -> (66.5817, -14.6605) centre (58.1002, -14.1001) ccw projected
  arc A17 (67.2926, -23.2925) -> (71.1002, -14.1001) centre (58.1002, -14.1001) ccw projected
  line L19 (71.1002, -14.1001) -> (71.1002, -5.7045) projected
  line L20 (71.1002, -5.7045) -> (68.1002, -5.7045) projected
  arc A18 (6.3002, 49.1999) -> (9.3002, 52.1999) centre (6.3002, 52.1999) ccw projected
  arc A19 (11.7898, 58.2103) -> (9.3002, 52.1999) centre (17.8002, 52.1999) ccw projected
  line L21 (11.7898, 58.2103) -> (31.9398, 78.3603) projected
  arc A20 (43.9606, 78.3603) -> (31.9398, 78.3603) centre (37.9502, 72.3499) ccw projected
  line L22 (43.9606, 78.3603) -> (64.1106, 58.2103) projected
  arc A21 (66.8919, 51.6165) -> (64.1106, 58.2103) centre (57.0713, 51.3576) ccw projected
  line L23 (66.8919, 51.6165) -> (68.1002, 49.1999) projected
  line L24 (68.1002, 49.1999) -> (68.1002, 37.9894) projected
  line L25 (68.1002, 37.9894) -> (71.1002, 37.9894) projected
  line L26 (71.1002, 37.9894) -> (71.1002, 52.1999) projected
  arc A22 (71.1002, 52.1999) -> (67.2926, 61.3923) centre (58.1002, 52.1999) ccw projected
  line L27 (67.2926, 61.3923) -> (47.1426, 81.5423) projected
  arc A23 (47.1426, 81.5423) -> (28.7578, 81.5423) centre (37.9502, 72.3499) ccw projected
  line L28 (28.7578, 81.5423) -> (8.6078, 61.3923) projected
  arc A24 (8.6078, 61.3923) -> (5.0308, 54.6374) centre (17.8002, 52.1999) ccw projected
  arc A25 (2.084, 52.1999) -> (5.0308, 54.6374) centre (2.084, 55.1999) ccw projected
  constraints: 2 end point, 1 vertical
extrude "Extrusion6" add sketch "Sketch8" along normal blind 3 contours A15 A14 L16 A13 L15 A16 L18 L17 L20 L19 A17 L14 A12 L13 A11 A10 L12 A6 L8 A5 L7 A4 L11 A25 A24 L28 A23 L27 A22 L26 L25 L24 L23 A21 L22 A20 L21 A19 A18 L10 A3 L6 A7 L5 A2 L4 A1 L3 A0 L2 A9 L1 A8 L0
sketch "Sketch10" plane through (-66.1, -12.6, -7.6) normal (0, -1, 0) x (1, 0, 0)
  line L0 (70.1002, -6.0043) -> (70.1002, -21.9894)
  arc A0 (67.2926, -61.3923) -> (71.1002, -52.1999) centre (58.1002, -52.1999) ccw construction
  line L1 (71.1002, -37.9894) -> (71.1002, -52.1999) construction
  line L2 (47.1426, -81.5423) -> (67.2926, -61.3923) construction
  line L3 (67.2926, -61.3923) -> (47.1426, -81.5423) construction
  arc A1 (5.0308, -54.6374) -> (8.6078, -61.3923) centre (17.8002, -52.1999) ccw construction
  line L4 (8.6078, -61.3923) -> (28.7578, -81.5423) construction
  line L5 (-68.9958, -52.1999) -> (2.084, -52.1999) construction
  line L6 (2.084, -52.1999) -> (-68.9958, -52.1999) construction
  line L7 (-98.3382, -28.2423) -> (-78.1882, -48.3923) construction
  line L8 (-78.1882, -48.3923) -> (-98.3382, -28.2423) construction
  arc A2 (-98.3382, -9.8575) -> (-98.3382, -28.2423) centre (-89.1458, -19.0499) ccw construction
  line L9 (-98.3382, -9.8575) -> (-78.1882, 10.2925) construction
  line L10 (2.084, 14.1001) -> (-68.9958, 14.1001) construction
  line L11 (-68.9958, 14.1001) -> (2.084, 14.1001) construction
  arc A3 (8.6078, 23.2925) -> (5.0308, 16.5376) centre (17.8002, 14.1001) ccw construction
  line L12 (8.6078, 23.2925) -> (28.7578, 43.4425) construction
  arc A4 (71.1002, 14.1001) -> (67.2926, 23.2925) centre (58.1002, 14.1001) ccw construction
  line L13 (47.1426, 43.4425) -> (67.2926, 23.2925) construction
  line L14 (71.1002, 14.1001) -> (71.1002, 5.7045) construction
  arc A5 (-98.3382, -9.8575) -> (-98.3382, -28.2423) centre (-89.1458, -19.0499) ccw construction
  arc A6 (-78.1882, -48.3923) -> (-68.9958, -52.1999) centre (-68.9958, -39.1999) ccw construction
  arc A7 (-78.1882, -48.3923) -> (-68.9958, -52.1999) centre (-68.9958, -39.1999) ccw construction
  arc A8 (-68.9958, 14.1001) -> (-78.1882, 10.2925) centre (-68.9958, 1.1001) ccw construction
  arc A9 (2.084, 14.1001) -> (5.0308, 16.5376) centre (2.084, 17.1001) ccw construction
  arc A10 (2.084, 14.1001) -> (2.084, 14.1001) centre (2.084, 17.1001) ccw construction
  arc A11 (5.0308, -54.6374) -> (2.084, -52.1999) centre (2.084, -55.1999) ccw construction
  arc A12 (2.084, 14.1001) -> (5.0308, 16.5376) centre (2.084, 17.1001) ccw construction
  arc A13 (5.0308, -54.6374) -> (8.6078, -61.3923) centre (17.8002, -52.1999) ccw construction
  arc A14 (8.6078, 23.2925) -> (5.0308, 16.5376) centre (17.8002, 14.1001) ccw construction
  line L15 (8.6078, -61.3923) -> (28.7578, -81.5423) construction
  arc A15 (28.7578, -81.5423) -> (47.1426, -81.5423) centre (37.9502, -72.3499) ccw construction
  arc A16 (67.2926, -61.3923) -> (71.1002, -52.1999) centre (58.1002, -52.1999) ccw construction
  arc A17 (71.1002, 14.1001) -> (67.2926, 23.2925) centre (58.1002, 14.1001) ccw construction
  arc A18 (47.1426, 43.4425) -> (28.7578, 43.4425) centre (37.9502, 34.2501) ccw construction
  arc A19 (47.1426, 43.4425) -> (28.7578, 43.4425) centre (37.9502, 34.2501) ccw construction
  line L16 (70.1002, -37.9894) -> (70.1002, -52.1999) construction
  arc A20 (66.5855, -60.6852) -> (70.1002, -52.1999) centre (58.1002, -52.1999) ccw construction
  line L17 (66.5855, -60.6852) -> (46.4355, -80.8352) construction
  arc A21 (29.4649, -80.8352) -> (46.4355, -80.8352) centre (37.9502, -72.3499) ccw construction
  line L18 (29.4649, -80.8352) -> (9.3149, -60.6852) construction
  arc A22 (6.0131, -54.4499) -> (9.3149, -60.6852) centre (17.8002, -52.1999) ccw construction
  arc A23 (6.0131, -54.4499) -> (2.084, -51.1999) centre (2.084, -55.1999) ccw construction
  line L19 (2.084, -51.1999) -> (-68.9958, -51.1999) construction
  arc A24 (-77.481, -47.6852) -> (-68.9958, -51.1999) centre (-68.9958, -39.1999) ccw construction
  line L20 (-77.481, -47.6852) -> (-97.6311, -27.5352) construction
  arc A25 (-97.6311, -10.5646) -> (-97.6311, -27.5352) centre (-89.1458, -19.0499) ccw construction
  line L21 (-97.6311, -10.5646) -> (-77.4811, 9.5854) construction
  arc A26 (-68.9958, 13.1001) -> (-77.4811, 9.5854) centre (-68.9958, 1.1001) ccw construction
  line L22 (-68.9958, 13.1001) -> (2.084, 13.1001) construction
  line L23 (70.1002, 5.7045) -> (70.1002, 14.1001) construction
  arc A27 (70.1002, 14.1001) -> (66.5855, 22.5854) centre (58.1002, 14.1001) ccw construction
  line L24 (66.5855, 22.5854) -> (46.4355, 42.7354) construction
  arc A28 (46.4355, 42.7354) -> (29.4649, 42.7354) centre (37.9502, 34.2501) ccw construction
  line L25 (29.4649, 42.7354) -> (9.3149, 22.5854) construction
  arc A29 (9.3149, 22.5854) -> (6.0131, 16.3501) centre (17.8002, 14.1001) ccw construction
  arc A30 (2.084, 13.1001) -> (6.0131, 16.3501) centre (2.084, 17.1001) ccw construction
  line L26 (70.1002, 5.7045) -> (71.1002, 5.7045) construction
  line L27 (68.1002, 10.3919) -> (68.1002, 5.7045) construction
  line L28 (70.1002, -37.9894) -> (71.1002, -37.9894) construction
  line L29 (70.1002, -6.0043) -> (71.1002, -6.0043)
  line L30 (71.1002, -21.9894) -> (71.1002, -6.0043) projected
  line L31 (71.1002, -6.0043) -> (71.1002, -21.9894)
  line L32 (71.1002, -21.9894) -> (70.1002, -21.9894)
  line L33 (70.1002, 14.1001) -> (70.1002, 5.7045)
  line L34 (68.1002, 5.7045) -> (71.1002, 5.7045) projected
  line L35 (71.1002, 5.7045) -> (70.1002, 5.7045)
  line L36 (71.1002, 5.7045) -> (71.1002, 14.1001)
  line L37 (66.5855, 22.5854) -> (46.4355, 42.7354)
  line L38 (47.1426, 43.4425) -> (67.2926, 23.2925)
  line L39 (29.4649, 42.7354) -> (9.3149, 22.5854)
  line L40 (28.7578, 43.4425) -> (8.6078, 23.2925)
  line L41 (2.084, 14.1001) -> (-68.9958, 14.1001)
  line L42 (-68.9958, 13.1001) -> (2.084, 13.1001)
  arc A31 (2.084, 14.1001) -> (5.0308, 16.5376) centre (2.084, 17.1001) ccw projected
  arc A32 (2.084, 14.1001) -> (5.0308, 16.5376) centre (2.084, 17.1001) ccw
  arc A33 (8.6078, 23.2925) -> (5.0308, 16.5376) centre (17.8002, 14.1001) ccw
  arc A34 (2.084, 13.1001) -> (6.0131, 16.3501) centre (2.084, 17.1001) ccw
  arc A35 (9.3149, 22.5854) -> (6.0131, 16.3501) centre (17.8002, 14.1001) ccw
  arc A36 (46.4355, 42.7354) -> (29.4649, 42.7354) centre (37.9502, 34.2501) ccw
  arc A37 (47.1426, 43.4425) -> (28.7578, 43.4425) centre (37.9502, 34.2501) ccw
  arc A38 (70.1002, 14.1001) -> (66.5855, 22.5854) centre (58.1002, 14.1001) ccw
  arc A39 (71.1002, 14.1001) -> (67.2926, 23.2925) centre (58.1002, 14.1001) ccw
  line L43 (70.1002, -52.1999) -> (70.1002, -37.9894)
  line L44 (70.1002, -37.9894) -> (71.1002, -37.9894)
  line L45 (71.1002, -52.1999) -> (71.1002, -37.9894) projected
  line L46 (66.5855, -60.6852) -> (46.4355, -80.8352)
  line L47 (47.1426, -81.5423) -> (67.2926, -61.3923)
  arc A40 (28.7578, -81.5423) -> (47.1426, -81.5423) centre (37.9502, -72.3499) ccw projected
  line L48 (29.4649, -80.8352) -> (9.3149, -60.6852)
  line L49 (8.6078, -61.3923) -> (28.7578, -81.5423)
  arc A41 (66.5855, -60.6852) -> (70.1002, -52.1999) centre (58.1002, -52.1999) ccw
  arc A42 (67.2926, -61.3923) -> (71.1002, -52.1999) centre (58.1002, -52.1999) ccw
  arc A43 (28.7578, -81.5423) -> (47.1426, -81.5423) centre (37.9502, -72.3499) ccw
  arc A44 (29.4649, -80.8352) -> (46.4355, -80.8352) centre (37.9502, -72.3499) ccw
  arc A45 (5.0308, -54.6374) -> (8.6078, -61.3923) centre (17.8002, -52.1999) ccw
  arc A46 (6.0131, -54.4499) -> (9.3149, -60.6852) centre (17.8002, -52.1999) ccw
  arc A47 (6.0131, -54.4499) -> (2.084, -51.1999) centre (2.084, -55.1999) ccw
  arc A48 (5.0308, -54.6374) -> (2.084, -52.1999) centre (2.084, -55.1999) ccw projected
  arc A49 (5.0308, -54.6374) -> (2.084, -52.1999) centre (2.084, -55.1999) ccw
  line L50 (2.084, -52.1999) -> (-68.9958, -52.1999)
  line L51 (-68.9958, -51.1999) -> (2.084, -51.1999)
  line L52 (-78.1882, -48.3923) -> (-98.3382, -28.2423) projected
  line L53 (-78.1882, -48.3923) -> (-98.3382, -28.2423)
  line L54 (-77.481, -47.6852) -> (-97.6311, -27.5352)
  arc A50 (-78.1882, -48.3923) -> (-68.9958, -52.1999) centre (-68.9958, -39.1999) ccw
  arc A51 (-77.481, -47.6852) -> (-68.9958, -51.1999) centre (-68.9958, -39.1999) ccw
  arc A52 (-97.6311, -10.5646) -> (-97.6311, -27.5352) centre (-89.1458, -19.0499) ccw
  arc A53 (-98.3382, -9.8575) -> (-98.3382, -28.2423) centre (-89.1458, -19.0499) ccw
  arc A54 (-68.9958, 13.1001) -> (-77.4811, 9.5854) centre (-68.9958, 1.1001) ccw
  arc A55 (-68.9958, 14.1001) -> (-78.1882, 10.2925) centre (-68.9958, 1.1001) ccw projected
  arc A56 (-68.9958, 14.1001) -> (-78.1882, 10.2925) centre (-68.9958, 1.1001) ccw
  line L55 (-97.6311, -10.5646) -> (-77.4811, 9.5854)
  line L56 (-78.1882, 10.2925) -> (-98.3382, -9.8575)
  point P0 (66.1, 7.6)
  dimension "d273" = 1
  dimension "d274" = 1
  constraints: 94 end point, 90 point on circle, 44 centre point, 18 tangent, 9 collinear, 8 perpendicular, 5 parallel, 4 horizontal, 2 concentric, 2 vertical, 1 vertical alignment, 22 other
  measures "d273" distance between parallel lines of L1 L16
  measures "d274" distance between parallel lines of L12 L25
extrude "Extrusion8" add sketch "Sketch10" along normal blind 1
sketch "Sketch19" plane through (-66.1, 7.69, -7.6) normal (0, 1, 0) x (1, 0, 0)
  line L0 (71.1002, -5.7045) -> (68.1002, -5.7045) projected
  line L1 (68.1002, 49.1999) -> (68.1002, 37.9894) projected
  line L2 (71.1002, -5.7045) -> (68.1002, -5.7045)
  line L3 (68.1002, -5.7045) -> (68.1002, 37.9894)
  line L4 (68.1002, 37.9894) -> (71.1002, 37.9894)
  line L5 (71.1002, 37.9894) -> (71.1002, -5.7045)
  point P0 (66.1, -7.6)
  constraints: 8 end point, 2 parallel, 1 horizontal, 1 perpendicular
extrude "Extrusion14" add sketch "Sketch19" against normal blind 3
sketch "Sketch13" plane through (-66.1, -12.6, -7.6) normal (0, -1, 0) x (1, 0, 0)
  line L0 (-91.4374, -10.2123) -> (-91.4374, -27.8875)
  line L1 (-92.3791, -9.2706) -> (-97.6458, -14.5373)
  line L2 (-97.6458, -14.5373) -> (-97.6458, -23.7339)
  line L3 (-97.6458, -23.7339) -> (-91.4374, -29.9423)
  line L4 (-91.4374, -29.9423) -> (-91.4374, -27.8875)
  circle A0 centre (-95.1541, -19.0499) radius 1.6
  arc A1 (-95.1562, -13.0395) -> (-95.1562, -25.0603) centre (-89.1458, -19.0499) ccw construction
  line L5 (-97.6458, -19.0499) -> (-109.6779, -19.0499) construction
  line L6 (-82.9257, -9.0889) -> (-87.7423, -9.0889) construction
  line L7 (-84.5257, -9.0889) -> (-86.6689, -9.0889) construction
  arc A2 (-98.3382, -9.8575) -> (-98.3382, -28.2423) centre (-89.1458, -19.0499) ccw projected
  line L8 (-91.4374, -19.0499) -> (-96.7541, -19.0499) construction
  line L9 (-97.6458, -19.0499) -> (-113.366, -19.0499) construction
  line L10 (-97.6458, -19.0499) -> (-100.3443, -19.0499)
  line L11 (-91.4374, -10.2123) -> (-91.4374, -8.3289)
  line L12 (-91.4374, -8.3289) -> (-92.3791, -9.2706)
  dimension "d209" = 3.2
  constraints: 26 end point, 6 point on line, 3 horizontal, 3 vertical, 1 horizontal alignment, 1 midpoint, 1 parallel, 1 point on circle, 2 other
extrude "Extrusion9" add sketch "Sketch13" against normal blind 20
sketch "Sketch14" plane through (2.0002, -12.6, -29.5894) normal (-1, 0, 0) x (0, 0, 1)
  line L0 (15.9851, 17.29) -> (15.9851, 0) construction
  line L1 (0, 17.29) -> (0, 0) construction
  line L2 (0, 0) -> (15.9851, 0) construction
  line L3 (7.9925, 0) -> (7.9925, 3) construction
  line L4 (7.9925, 3) -> (15.9851, 3) construction
  line L5 (15.9851, 3) -> (15.9851, 5) construction
  line L6 (15.9851, 17.29) -> (15.9851, 0) construction
  line L7 (15.9851, 5) -> (0, 8.145) construction
  line L8 (15.9851, 3) -> (0, 3)
  line L9 (0, 3) -> (0, 8.145)
  line L10 (0, 8.145) -> (15.9851, 8.145)
  line L11 (15.9851, 8.145) -> (15.9851, 3)
  point P0 (29.5894, 12.6)
  point P1 (15.9851, 11)
  point P2 (15.9851, -1)
  point P3 (0, 11)
  point P4 (0, -1)
  dimension "d210" = 3
  dimension "d211" = 2
  constraints: 16 end point, 3 point on line, 2 parallel, 2 perpendicular, 1 horizontal, 1 midpoint, 1 vertical
  measures "d210" distance of L3.start L3.end
  measures "d211" distance of L4.end L5.end
extrude "Extrusion10" cut sketch "Sketch14" against normal blind 1
sketch "Sketch15" plane through (-157.5374, -12.6, -17.8123) normal (1, 0, 0) x (0, 0, -1)
  line L0 (18.5668, 0) -> (-0.8917, 0) construction
  line L1 (8.8376, 0) -> (8.8376, 3) construction
  line L2 (8.8376, 0) -> (11.8376, 0) construction
  line L3 (8.8376, 3) -> (0, 3) construction
  line L4 (0, 3) -> (0, 5) construction
  line L5 (0, 0) -> (0, 17.29) construction
  line L6 (0, 5) -> (17.6751, 5) construction
  line L7 (17.6751, 17.29) -> (17.6751, 0) construction
  line L8 (0, 3) -> (17.6751, 3)
  line L9 (17.6751, 3) -> (17.6751, 5)
  line L10 (17.6751, 5) -> (0, 5)
  line L11 (0, 5) -> (0, 3)
  line L12 (-0.8917, 20) -> (18.5668, 20) projected
  line L13 (18.5668, 20) -> (18.5668, 0) projected
  line L14 (-0.8917, 0) -> (-0.8917, 20) projected
  point P0 (-17.8123, 12.6)
  dimension "d214" = 3
  dimension "d215" = 90
  dimension "d216" = 2
  constraints: 18 end point, 4 perpendicular, 2 horizontal, 2 parallel, 2 point on line, 1 midpoint, 1 vertical
  measures "d214" distance of L1.start L1.end
  measures "d215" angle of L2 L1
  measures "d216" distance of L3.end L4.end
extrude "Extrusion11" cut sketch "Sketch15" against normal blind 1
sketch "Sketch18" plane through (-64.016, 4.69, -59.7999) normal (0, 0, -1) x (-1, 0, 0)
  line L0 (44.1622, -18.29) -> (71.0798, -18.29) construction
  line L1 (71.0798, -18.29) -> (71.0798, -1) construction
  line L2 (71.0798, -1) -> (44.1622, -1) construction
  line L3 (44.1622, -1) -> (44.1622, -18.29) construction
  line L4 (71.0798, -1) -> (71.0798, -18.29) construction
  line L5 (71.0798, -9.645) -> (44.1622, -9.645) construction
  line L6 (44.1622, -1) -> (44.1622, -18.29) construction
  arc A0 (55.5252, -6.11) -> (61.6635, -6.11) centre (58.5944, -10) ccw
  line L7 (55.5252, -6.11) -> (61.6635, -6.11)
  line L8 (50.344, -9.645) -> (54.4692, -2.5) construction
  line L9 (54.4692, -2.5) -> (62.7195, -2.5) construction
  line L10 (62.7195, -2.5) -> (66.8447, -9.645) construction
  line L11 (66.8447, -9.645) -> (62.7195, -16.79) construction
  line L12 (62.7195, -16.79) -> (54.4692, -16.79) construction
  line L13 (54.4692, -16.79) -> (50.344, -9.645) construction
  line L14 (58.5944, -9.645) -> (54.4692, -2.5) construction
  line L15 (58.5944, -10) -> (58.5944, -1.75) construction
  line L16 (-36.0162, -1) -> (71.0798, -1) construction
  line L17 (58.5944, -9) -> (66.8444, -9) construction
  line L18 (58.5944, -1) -> (58.5944, -0.8021) construction
  line L19 (58.5944, -9) -> (58.5944, -10) construction
  line L20 (58.5944, -9) -> (59.5944, -9) construction
  line L21 (44.5764, -17.29) -> (44.5764, 3) projected
  line L22 (71.0798, -17.29) -> (71.0798, 3) projected
  line L23 (44.5764, 3) -> (71.0798, 3) projected
  line L24 (71.0798, -17.29) -> (44.5764, -17.29) projected
  point P0 (-64.016, -4.69)
  point P1 (5.0002, -4.69)
  dimension "d253" = 9.91
  dimension "d254" = 14.29
  dimension "d255" = 8.2503
  dimension "d256" = 8.25
  dimension "d257" = 90
  dimension "d258" = 0.75
  dimension "d259" = 1
  dimension "d260" = 90
  dimension "d261" = 6.1818
  constraints: 42 end point, 4 horizontal, 4 perpendicular, 2 midpoint, 2 parallel, 2 point on circle, 2 point on line, 1 centre point, 1 coincident, 1 vertical
  measures "d253" diameter of A0
  measures "d254" distance between parallel lines of L9 L12
  measures "d255" distance of L14.start L8.end
  measures "d256" distance of L15.start L15.end
  measures "d257" angle of L17 L15
  measures "d258" distance of L15.end L18.start
  measures "d259" distance of L19.start L19.end
  measures "d260" angle of L19 L20
  measures "d261" distance from line of L3 L8.start
extrude "Extrusion13" cut sketch "Sketch18" against normal blind 100 contours L7 A0